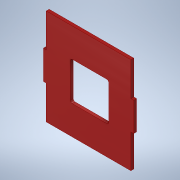
# Autodesk Inventor part: Part3
Saved by Autodesk Inventor 2020 (Build 240168000, 168)
## iProperties
Created: 2020-03-09
Part Number: Part3
Material: Generic
Document SubType Name: Modeling
Designer: tor16003
Density: 1 g/cm^3
Appearance: Red
Author: tor16003
Autodesk Inventor part; units mm, degrees
ref_plane "YZ Plane" through (0, 0, 0) normal (1, 0, 0) x (0, 1, 0)
ref_plane "XZ Plane" through (0, 0, 0) normal (0, 1, 0) x (-1, 0, 0)
ref_plane "XY Plane" through (0, 0, 0) normal (0, 0, 1) x (1, 0, 0)
sketch "Sketch1" plane through (0, 0, 0) normal (0, 0, 1) x (1, 0, 0)
  line L0 (-3, 35) -> (0, 35)
  line L1 (-3, 35) -> (-3, 65)
  line L2 (-3, 65) -> (0, 65)
  line L3 (0, 65) -> (0, 100)
  line L4 (0, 100) -> (88, 100)
  line L5 (88, 100) -> (88, 65)
  line L6 (88, 65) -> (91, 65)
  line L7 (91, 65) -> (91, 35)
  line L8 (91, 35) -> (88, 35)
  line L9 (88, 35) -> (88, 0)
  line L10 (88, 0) -> (0, 0)
  line L11 (0, 0) -> (0, 35)
  line L12 (63, 70) -> (27, 70)
  line L13 (25, 68) -> (25, 32)
  line L14 (27, 30) -> (63, 30)
  line L15 (65, 32) -> (65, 68)
  arc A0 (65, 68) -> (63, 70) centre (63, 68) ccw
  arc A1 (63, 30) -> (65, 32) centre (63, 32) ccw
  arc A2 (25, 32) -> (27, 30) centre (27, 32) ccw
  arc A3 (27, 70) -> (25, 68) centre (27, 68) ccw
  point P0 (25, 30)
  point P1 (25, 70)
  point P2 (65, 30)
  dimension "d0" = 3
  dimension "d10" = 30
  dimension "d21" = 35
  dimension "d22" = 100
  dimension "d30" = 88
  dimension "d32" = 3
  dimension "d40" = 40
  dimension "d41" = 40
  dimension "d42" = 2
  dimension "d43" = 30
  dimension "d44" = 25
  constraints: 32 end point, 8 perpendicular, 8 point on circle, 8 tangent, 6 point on line, 4 centre point, 4 horizontal, 4 parallel, 3 equal radius, 2 collinear, 1 coincident, 1 vertical
  measures "d0" distance of L0.start L0.end
  measures "d10" distance of L6.end L7.end
  measures "d21" distance of L8.end L9.end
  measures "d22" distance of L9.end L4.end
  measures "d30" distance between parallel lines of L11 L9
  measures "d32" distance between parallel lines of L5 L7
  measures "d40" distance of point (65, 30) point (25, 30)
  measures "d41" distance of point (25, 30) point (25, 70)
  measures "d42" radius of A0
  measures "d43" distance between parallel lines of L4 L12
  measures "d44" distance between parallel lines of L3 L13
extrude "Extrusión3" add sketch "Sketch1" along normal blind 3
